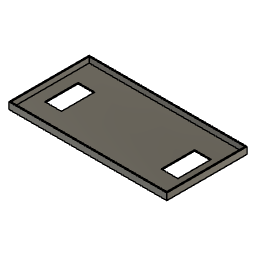
couvercle_boitier (Autodesk Fusion 360 design; units mm, degrees)
Autodesk Fusion 360 part; units mm, degrees
sketch "Esquisse1" plane through (0, 0, 0) normal (0, 0, 1) x (1, 0, 0)
  line L0 (71.2, 51.2) -> (-71.2, 51.2)
  line L1 (-71.2, 51.2) -> (-71.2, -21.2)
  line L2 (-71.2, -21.2) -> (71.2, -21.2)
  line L3 (71.2, -21.2) -> (71.2, 51.2)
  constraint horizontal L0
  constraint vertical L1
  constraint horizontal L2
  constraint vertical L3
extrude "Extrusion1" add sketch "Esquisse1" along normal blind 5
extrude "Extrusion2" add 1 faces at (-23.7333, 27.0667, 5) along direction (0, 0, 1) blind 1
sketch "Esquisse2" plane through (0, 0, 6) normal (0, 0, 1) x (-1, 0, 0)
  line L0 (-71.2, 21.2) -> (-71.2, -51.2)
  line L1 (-71.2, -51.2) -> (71.2, -51.2)
  line L2 (71.2, -51.2) -> (71.2, 21.2)
  line L3 (71.2, 21.2) -> (-71.2, 21.2)
  line L4 (70.2, -50.2) -> (-70.2, -50.2)
  line L5 (-70.2, -50.2) -> (-70.2, 20.2)
  line L6 (-70.2, 20.2) -> (70.2, 20.2)
  line L7 (70.2, 20.2) -> (70.2, -50.2)
  constraint horizontal L4
  constraint vertical L5
  constraint horizontal L6
  constraint vertical L7
extrude "Extrusion3" cut sketch "Esquisse2" against normal blind 5 contours L4 L5 L6 L7
sketch "Esquisse3" plane through (0, 0, 1) normal (0, 0, 1) x (-1, 0, 0)
  line L0 (70.2, 20.2) -> (-70.2, 20.2)
  line L1 (-70.2, 20.2) -> (-70.2, -50.2)
  line L2 (-70.2, -50.2) -> (70.2, -50.2)
  line L3 (70.2, -50.2) -> (70.2, 20.2)
  line L4 (45, 0) -> (60, 0)
  line L5 (60, 0) -> (60, -30)
  line L6 (60, -30) -> (45, -30)
  line L7 (45, -30) -> (45, 0)
  line L8 (-60, 0) -> (-45, 0)
  line L9 (-45, 0) -> (-45, -30)
  line L10 (-45, -30) -> (-60, -30)
  line L11 (-60, -30) -> (-60, 0)
  constraint horizontal L4
  constraint vertical L5
  constraint horizontal L6
  constraint vertical L7
  constraint horizontal L8
  constraint vertical L9
  constraint horizontal L10
  constraint vertical L11
extrude "Extrusion4" cut sketch "Esquisse3" against normal blind 1 contours L4 L5 L6 L7 | L8 L9 L10 L11
